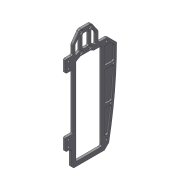
# Autodesk Inventor part: VerticalFrame
Saved by Autodesk Inventor 2019.4 (Build 234330000, 330)
## iProperties
Created: 2019-01-12
Part Number: VerticalFrame
Material: 一般
Document SubType Name: Modeling
Designer: y6tada
Density: 1 g/cm^3
Appearance: 既定
Mass: 8.8829 g
Surface Area: 108.713 cm^2
Volume: 8.8829 cm^3
Author: y6tada
Autodesk Inventor part; units mm, degrees
ref_plane "YZ Plane" through (0, 0, 0) normal (1, 0, 0) x (0, 1, 0)
ref_plane "XZ Plane" through (0, 0, 0) normal (0, 1, 0) x (-1, 0, 0)
ref_plane "XY Plane" through (0, 0, 0) normal (0, 0, 1) x (1, 0, 0)
sketch "スケッチ1" plane through (0, 0, 0) normal (1, 0, 0) x (0, 1, 0)
  line L0 (32, 59) -> (0.2256, 59) construction
  line L1 (-1, 56.6671) -> (-1, -58)
  line L2 (0, -59) -> (32, -59)
  line L3 (34, -57) -> (34, 57)
  line L4 (-7, 67) -> (-14, 67)
  line L5 (-15, 66) -> (-15, 51.5)
  line L6 (-14, 50.5) -> (-6, 50.5)
  line L7 (-5, 49.5) -> (-5, -23.5)
  line L8 (-6, -24.5) -> (-14, -24.5)
  line L9 (-15, -25.5) -> (-15, -40)
  line L10 (-14, -41) -> (-10, -41)
  line L11 (-4, -65) -> (37.454, -65)
  line L12 (18, 92.25) -> (6, 92.25)
  line L13 (0, 0) -> (34, 0) construction
  line L14 (-7, -62) -> (-4, -65)
  line L15 (31, 65) -> (40.3431, 65)
  circle A0 centre (-11, 63) radius 1.3
  circle A1 centre (-11, 54.5) radius 1.3
  circle A2 centre (-11, -28.5) radius 1.3
  circle A3 centre (-11, -37) radius 1.3
  line L16 (-11, 63) -> (-11, 54.5) construction
  line L17 (-11, -28.5) -> (-11, -37) construction
  circle A4 centre (18, 88.75) radius 1.05 construction
  circle A5 centre (6, 88.75) radius 1.05 construction
  circle A6 centre (6, 64.75) radius 1.05 construction
  circle A7 centre (18, 64.75) radius 1.05 construction
  circle A8 centre (18, 88.75) radius 1.3
  circle A9 centre (6, 88.75) radius 1.3
  circle A10 centre (6, 64.75) radius 1.3
  circle A11 centre (18, 64.75) radius 1.3
  arc A12 (20.867, 90.7575) -> (18, 92.25) centre (18, 88.75) ccw
  arc A13 (6, 92.25) -> (3.133, 90.7575) centre (6, 88.75) ccw
  line L18 (-7, -44) -> (-7, -62)
  arc A14 (-7, -44) -> (-10, -41) centre (-10, -44) ccw
  arc A15 (34, 57) -> (32, 59) centre (32, 57) ccw
  arc A16 (32, -59) -> (34, -57) centre (32, -57) ccw
  line L19 (43.1716, 63.8284) -> (54, 53)
  arc A17 (43.454, -59) -> (54, 53) centre (-546, 53) ccw
  line L20 (54, 80.46) -> (54, 17.89) construction
  arc A18 (-1, -58) -> (0, -59) centre (0, -58) ccw
  arc A19 (43.1716, 63.8284) -> (40.3431, 65) centre (40.3431, 61) ccw
  line L21 (20.867, 90.7575) -> (28.367, 80.0464)
  line L22 (29, 78.0389) -> (29, 67)
  line L23 (3.133, 90.7575) -> (-4.367, 80.0464)
  line L24 (-5, 78.0389) -> (-5, 69)
  line L25 (12, 92.25) -> (12, 64.3882) construction
  arc A20 (29, 78.0389) -> (28.367, 80.0464) centre (25.5, 78.0389) ccw
  arc A21 (-4.367, 80.0464) -> (-5, 78.0389) centre (-1.5, 78.0389) ccw
  arc A22 (29, 67) -> (31, 65) centre (31, 67) ccw
  arc A23 (-7, 67) -> (-5, 69) centre (-7, 69) ccw
  line L26 (14.5, 86.25) -> (9.5, 86.25)
  line L27 (7.5, 84.25) -> (7.5, 69.75)
  line L28 (9.5, 67.75) -> (14.5, 67.75)
  line L29 (16.5, 69.75) -> (16.5, 84.25)
  arc A24 (16.5, 84.25) -> (14.5, 86.25) centre (14.5, 84.25) ccw
  arc A25 (14.5, 67.75) -> (16.5, 69.75) centre (14.5, 69.75) ccw
  arc A26 (7.5, 69.75) -> (9.5, 67.75) centre (9.5, 69.75) ccw
  arc A27 (9.5, 86.25) -> (7.5, 84.25) centre (9.5, 84.25) ccw
  line L30 (19.5, 84.3079) -> (19.5, 68.5028)
  line L31 (20, 67.6368) -> (24.5, 65.0387)
  line L32 (26, 65.9047) -> (26, 77.8812)
  line L33 (25.8192, 78.4548) -> (21.3192, 84.8815)
  arc A28 (24.5, 65.0387) -> (26, 65.9047) centre (25, 65.9047) ccw
  arc A29 (19.5, 68.5028) -> (20, 67.6368) centre (20.5, 68.5028) ccw
  arc A30 (21.3192, 84.8815) -> (19.5, 84.3079) centre (20.5, 84.3079) ccw
  arc A31 (26, 77.8812) -> (25.8192, 78.4548) centre (25, 77.8812) ccw
  line L34 (4.5, 84.3079) -> (4.5, 68.5028)
  line L35 (4, 67.6368) -> (-0.5, 65.0387)
  line L36 (-2, 65.9047) -> (-2, 77.8812)
  line L37 (-1.8192, 78.4548) -> (2.6808, 84.8815)
  arc A32 (-2, 65.9047) -> (-0.5, 65.0387) centre (-1, 65.9047) ccw
  arc A33 (4, 67.6368) -> (4.5, 68.5028) centre (3.5, 68.5028) ccw
  arc A34 (4.5, 84.3079) -> (2.6808, 84.8815) centre (3.5, 84.3079) ccw
  arc A35 (-1.8192, 78.4548) -> (-2, 77.8812) centre (-1, 77.8812) ccw
  arc A36 (-5, 49.5) -> (-6, 50.5) centre (-6, 49.5) ccw
  arc A37 (-6, -24.5) -> (-5, -23.5) centre (-6, -23.5) ccw
  line L38 (-14, 67) -> (-15, 66)
  line L39 (-15, 51.5) -> (-14, 50.5)
  line L40 (-14, -24.5) -> (-15, -25.5)
  line L41 (-15, -40) -> (-14, -41)
  circle A38 centre (40.3431, 61) radius 1.3
  line L42 (54, 53) -> (-546, 53) construction
  line L43 (37.454, -65) -> (43.454, -59)
  arc A39 (39.0418, -60.7632) -> (49.9964, 55.0735) centre (-546, 53) ccw construction
  circle A40 centre (49.5938, 31) radius 1.3
  circle A41 centre (46.2221, -14) radius 1.3
  circle A42 centre (40.3165, -54) radius 1.3
  line L44 (22.4952, 59.2679) -> (19.5263, 60.9821)
  line L45 (18.5263, 61.25) -> (5.4737, 61.25)
  line L46 (4.4737, 60.9821) -> (0, 58.3991)
  line L47 (32, 59) -> (23.4952, 59)
  arc A43 (22.4952, 59.2679) -> (23.4952, 59) centre (23.4952, 61) ccw
  arc A44 (19.5263, 60.9821) -> (18.5263, 61.25) centre (18.5263, 59.25) ccw
  arc A45 (5.4737, 61.25) -> (4.4737, 60.9821) centre (5.4737, 59.25) ccw
  arc A46 (0, 58.3991) -> (-1, 56.6671) centre (1, 56.6671) ccw
  point P0 (34, 59)
  point P1 (-1, -59)
  point P2 (-1, 59)
  point P3 (34, -59)
  point P4 (-23.0245, 67)
  point P5 (-15, 67)
  point P6 (-15, 50.5)
  point P7 (-5, 50.5)
  point P8 (-5, -24.5)
  point P9 (-15, -24.5)
  point P10 (-15, -41)
  point P11 (-5, -41)
  point P12 (2.5, 68.5585)
  point P13 (42, 65)
  point P14 (24.5, 65)
  point P15 (-13.5, 67)
  point P16 (-1, 57.9118)
  point P17 (-1.5, 78.0389)
  point P18 (22.9593, 59)
  dimension "d2" = 118
  dimension "d4" = 108
  dimension "d5" = 16.5
  dimension "d6" = 16.5
  dimension "d7" = 4
  dimension "d8" = 2.6
  dimension "d10" = 4
  dimension "d11" = 4
  dimension "d12" = 4
  dimension "d13" = 4
  dimension "d14" = 4
  dimension "d15" = 4
  dimension "d16" = 10
  dimension "d17" = 2.6
  dimension "d18" = 3.5
  dimension "d20" = 35
  dimension "d21" = 3
  dimension "d22" = 6
  dimension "d24" = 2
  dimension "d26" = 45
  dimension "d27" = 600
  dimension "d28" = 20
  dimension "d29" = 6
  dimension "d30" = 45
  dimension "d32" = 3
  dimension "d33" = 1
  dimension "d36" = 4
  dimension "d37" = 35
  dimension "d38" = 35
  dimension "d39" = 34
  dimension "d40" = 3.5
  dimension "d41" = 2
  dimension "d42" = 6
  dimension "d43" = 3
  dimension "d44" = 9
  dimension "d45" = 2
  dimension "d46" = 1
  dimension "d47" = 3
  dimension "d48" = 3
  dimension "d49" = 3
  dimension "d50" = 3.5
  dimension "d51" = 1
  dimension "d52" = 1
  dimension "d53" = 45
  dimension "d54" = 1
  dimension "d55" = 45
  dimension "d56" = 1
  dimension "d57" = 45
  dimension "d58" = 1
  dimension "d59" = 45
  dimension "d60" = 45
  dimension "d61" = 6
  dimension "d62" = 4
  dimension "d63" = 30
  dimension "d64" = 45
  dimension "d65" = 40
  dimension "d69" = 120
  dimension "d70" = 6
  dimension "d71" = 6.5
  dimension "d72" = 6
  dimension "d73" = 6
  dimension "d74" = 2
  dimension "d93" = 12
  dimension "d95" = 11
  constraints: 96 end point, 65 point on circle, 51 tangent, 43 centre point, 31 point on line, 24 equal radius, 13 symmetric about line, 10 parallel, 9 perpendicular, 7 vertical, 6 horizontal, 5 coincident, 2 collinear, 2 concentric, 2 midpoint, 6 other
  measures "d2" distance of point (34, -59) point (34, 59)
  measures "d4" distance between parallel lines of L4 L10
  measures "d5" distance of point (-15, -24.5) point (-15, -41)
  measures "d6" distance of point (-15, 67) point (-15, 50.5)
  measures "d7" distance from line of L17.start L8
  measures "d8" diameter of A2
  measures "d10" distance from line of L10 L17.end
  measures "d11" distance between parallel lines of L5 L16
  measures "d12" distance from line of L6 L16.end
  measures "d13" distance from line of L4 L16.start
  measures "d14" distance between parallel lines of L17 L9
  measures "d15" distance between parallel lines of L1 L7
  measures "d16" distance of point (-15, 50.5) point (-5, 50.5)
  measures "d17" diameter of A8
  measures "d18" radius of A12
  measures "d20" distance of point (34, 59) point (-1, 59)
  measures "d21" radius of A14
  measures "d22" distance between parallel lines of L18 L1
  measures "d24" radius of A15
  measures "d26" angle of L19 L15
  measures "d27" radius of A17
  measures "d28" distance between parallel lines of L3 L20
  measures "d29" distance between parallel lines of L11 L2
  measures "d30" angle of L14 L18
  measures "d32" distance from line of L14.start L11
  measures "d33" radius of A18
  measures "d36" radius of A19
  measures "d37" angle of L22 L21
  measures "d38" angle of L24 L23
  measures "d39" distance between parallel lines of L24 L22
  measures "d40" radius of A20
  measures "d41" radius of A22
  measures "d42" distance between parallel lines of L26 L12
  measures "d43" distance from line of A7.centre L28
  measures "d44" distance between parallel lines of L27 L29
  measures "d45" radius of A24
  measures "d46" radius of A28
  measures "d47" distance between parallel lines of L22 L32
  measures "d48" distance between parallel lines of L21 L33
  measures "d49" distance between parallel lines of L29 L30
  measures "d50" distance from line of A7.centre L31
  measures "d51" radius of A36
  measures "d52" distance of L4.end point (-15, 67)
  measures "d53" angle of L4 L38
  measures "d54" distance of L5.end point (-15, 50.5)
  measures "d55" angle of L5 L39
  measures "d56" distance of L8.end point (-15, -24.5)
  measures "d57" angle of L8 L40
  measures "d58" distance of L9.end point (-15, -41)
  measures "d59" angle of L9 L41
  measures "d60" angle of L43 L11
  measures "d61" distance from line of L43.end L11
  measures "d62" radial gap between concentric circles of A39 A17
  measures "d63" vertical distance of A40.centre A19.centre
  measures "d64" vertical distance of A41.centre A40.centre
  measures "d65" vertical distance of A42.centre A41.centre
  measures "d69" angle of L30 L31
  measures "d70" distance between parallel lines of L0 L15
  measures "d71" distance between parallel lines of L28 L45
  measures "d72" distance between parallel lines of L31 L44
  measures "d73" distance between parallel lines of L35 L46
  measures "d74" radius of A43
  measures "d93" distance between parallel lines of L42 L15
  measures "d95" distance from line of L16 L13.start
extrude "押し出し1" add sketch "スケッチ1" along normal blind 3
sketch "スケッチ2" plane through (3, 0, 0) normal (1, 0, 0) x (0, 0, -1)
  circle A0 centre (-88.75, 18) radius 1.3 projected
  circle A1 centre (-88.75, 18) radius 2.5
  circle A2 centre (-88.75, 6) radius 1.3 projected
  circle A3 centre (-88.75, 6) radius 2.5
  circle A4 centre (-64.75, 6) radius 1.3 projected
  circle A5 centre (-64.75, 6) radius 2.5
  circle A6 centre (-64.75, 18) radius 1.3 projected
  circle A7 centre (-64.75, 18) radius 2.5
  point P0 (0, 0)
  dimension "d66" = 5
  constraints: 4 centre point, 4 coincident, 3 equal radius
  measures "d66" diameter of A1
extrude "押し出し2" cut sketch "スケッチ2" against normal blind 1.5
sketch "スケッチ3" plane through (3, 0, 0) normal (1, 0, 0) x (0, 0, -1)
  circle A0 centre (-31, 49.5938) radius 1.3 construction
  line L0 (-31, 49.5938) -> (-31.9952, 22.6513) construction
  circle A1 centre (14, 46.2221) radius 1.3 construction
  line L1 (14, 46.2221) -> (11.2386, 21.8138) construction
  arc A2 (11.2386, 21.8138) -> (11.2386, 21.8138) centre (23.9128, 20.3799) ccw
  line L2 (-53, 54) -> (-63.8284, 43.1716) construction
  arc A3 (59, 43.454) -> (-53, 54) centre (-53, -546) ccw construction
  line L3 (-57, 34) -> (57, 34) construction
  line L4 (-52.4939, 50.2634) -> (-56.2678, 46.4896)
  line L5 (-33.0546, 48.1516) -> (-33.3776, 39.4077)
  line L6 (-29.0574, 48.004) -> (-29.3681, 39.5923)
  line L7 (-57, 39.5) -> (-57, 44.7218)
  line L8 (11.8421, 44.9395) -> (11.195, 39.219)
  line L9 (15.8168, 44.4898) -> (15.2841, 39.781)
  circle A4 centre (54, 40.3165) radius 1.3 construction
  line L10 (54, 40.3165) -> (51.075, 24.2885) construction
  line L11 (48.8034, 39.6919) -> (48.6865, 39.0512)
  line L12 (-54.5, 37) -> (-35.8759, 37)
  line L13 (-26.8698, 37) -> (8.7108, 37)
  line L14 (17.7682, 37) -> (46.2271, 37)
  arc A5 (-35.4796, 50.7429) -> (-50.7166, 50.9956) centre (-53, -546) ccw
  arc A6 (-50.7166, 50.9956) -> (-52.4939, 50.2634) centre (-50.7262, 48.4957) ccw
  arc A7 (-33.0546, 48.1516) -> (-35.4796, 50.7429) centre (-35.5529, 48.2439) ccw
  arc A8 (-35.8759, 37) -> (-33.3776, 39.4077) centre (-35.8759, 39.5) ccw
  arc A9 (-57, 39.5) -> (-54.5, 37) centre (-54.5, 39.5) ccw
  arc A10 (-56.2678, 46.4896) -> (-57, 44.7218) centre (-54.5, 44.7218) ccw
  arc A11 (9.6202, 47.7068) -> (-26.4479, 50.4092) centre (-53, -546) ccw
  arc A12 (-26.4479, 50.4092) -> (-29.0574, 48.004) centre (-26.5591, 47.9117) ccw
  arc A13 (11.8421, 44.9395) -> (9.6202, 47.7068) centre (9.358, 45.2205) ccw
  arc A14 (8.7108, 37) -> (11.195, 39.219) centre (8.7108, 39.5) ccw
  arc A15 (-29.3681, 39.5923) -> (-26.8698, 37) centre (-26.8698, 39.5) ccw
  arc A16 (46.7618, 42.6056) -> (18.6008, 46.6908) centre (-53, -546) ccw
  arc A17 (18.6008, 46.6908) -> (15.8168, 44.4898) centre (18.3009, 44.2088) ccw
  arc A18 (48.8034, 39.6919) -> (46.7618, 42.6056) centre (46.3441, 40.1408) ccw
  arc A19 (46.2271, 37) -> (48.6865, 39.0512) centre (46.2271, 39.5) ccw
  arc A20 (15.2841, 39.781) -> (17.7682, 37) centre (17.7682, 39.5) ccw
  circle A21 centre (-61, 40.3431) radius 1.3 construction
  point P0 (0, 0)
  point P1 (-33.5774, 34)
  point P2 (-29.5746, 34)
  point P3 (10.6045, 34)
  point P4 (14.63, 34)
  point P5 (49.257, 42.1773)
  dimension "d76" = 3
  dimension "d78" = 2
  dimension "d79" = 2
  dimension "d80" = 2
  dimension "d81" = 2
  dimension "d82" = 2.5
  dimension "d83" = 3
  dimension "d84" = 2.5
  dimension "d85" = 3
  dimension "d86" = 2.5
  dimension "d87" = 3
  dimension "d88" = 3
  dimension "d89" = 4
  dimension "d90" = 5
  constraints: 35 point on circle, 27 tangent, 26 end point, 17 centre point, 13 point on line, 10 equal radius, 9 parallel, 2 collinear, 1 vertical
  measures "d76" distance between parallel lines of L2 L4
  measures "d78" distance between parallel lines of L0 L5
  measures "d79" distance between parallel lines of L6 L0
  measures "d80" distance between parallel lines of L1 L8
  measures "d81" distance between parallel lines of L1 L9
  measures "d82" radius of A6
  measures "d83" radial gap between concentric circles of A3 A11
  measures "d84" radius of A12
  measures "d85" radial gap between concentric circles of A3 A16
  measures "d86" radius of A17
  measures "d87" distance between parallel lines of L12 L3
  measures "d88" radial gap between concentric circles of A3 A5
  measures "d89" distance from line of L7 A21.centre
  measures "d90" distance between parallel lines of L10 L11
extrude "押し出し3" cut sketch "スケッチ3" against normal blind 2 contours A6 A5 A7 L5 A8 L12 A9 L7 A10 L4 | A12 A11 A13 L8 A14 L13 A15 L6 | A17 A16 A18 L11 A19 L14 A20 L9
